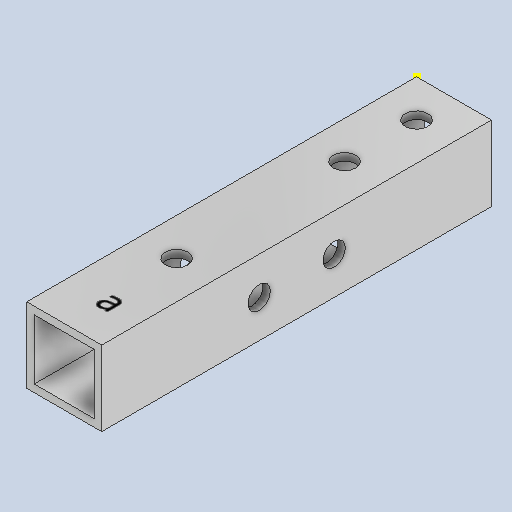
# Autodesk Inventor part: finger_k_mk_2
Saved by Autodesk Inventor 2024.1 (Build 281209000, 209)
## iProperties
Created: 2022-06-23
Part Number: finger_k_mk_2
Material: アルミニウム 6061-AHC
Document SubType Name: Modeling
Designer: zegi
Density: 2.7 g/cm^3
Appearance: アルミニウム - ダーク
Mass: 4.86355 g
Surface Area: 37.6888 cm^2
Volume: 1.80131 cm^3
Author: zegi
Autodesk Inventor part; units mm, degrees
ref_plane "YZ Plane" through (0, 0, 0) normal (1, 0, 0) x (0, 1, 0)
ref_plane "XZ Plane" through (0, 0, 0) normal (0, 1, 0) x (-1, 0, 0)
ref_plane "XY Plane" through (0, 0, 0) normal (0, 0, 1) x (1, 0, 0)
sketch "スケッチ1" plane through (0, 0, 0) normal (0, 0, 1) x (1, 0, 0)
  line L0 (0, 0) -> (10, 0)
  line L1 (10, 0) -> (10, 10)
  line L2 (10, 10) -> (0, 10)
  line L3 (0, 10) -> (0, 0)
  line L4 (1, 9) -> (9, 9)
  line L5 (9, 9) -> (9, 1)
  line L6 (9, 1) -> (1, 1)
  line L7 (1, 1) -> (1, 9)
  dimension "d0" = 10
  dimension "d1" = 10
  dimension "d2" = 1
  constraints: 16 end point, 4 parallel, 2 perpendicular, 1 horizontal, 3 other
  measures "d0" distance of L2.end L1.end
  measures "d1" distance of L1.end L0.end
  measures "d2" distance between parallel lines of L2 L4
extrude "押し出し1" add sketch "スケッチ1" along normal blind 52
sketch "スケッチ2" plane through (0, 10, 0) normal (0, 1, 0) x (1, 0, 0)
  line L0 (10, -52) -> (0, -52) projected
  line L1 (10, 0) -> (10, -52) projected
  line L2 (10, -26) -> (0, -26)
  line L3 (0, 0) -> (0, -52) projected
  point P0 (5, -37)
  point P1 (5, -14.6)
  point P2 (5, -5)
  dimension "d5" = 22.4
  dimension "d7" = 5
  dimension "d8" = 5
  dimension "d35" = 9.6
  dimension "d36" = 11
  constraints: 2 end point, 2 midpoint
  measures "d5" distance of point (5, -14.6) point (5, -37)
  measures "d7" distance from line of L1 point (5, -37)
  measures "d8" distance from line of L1 point (5, -14.6)
  measures "d35" distance of point (5, -5) point (5, -14.6)
  measures "d36" distance from line of L2 point (5, -37)
hole "穴1" at (5, 10, 37) at (5, 10, 14.6) at (5, 10, 5) direction (0, -1, 0) diameter 3 end through all
sketch "スケッチ3" plane through (10, 0, 0) normal (1, 0, 0) x (0, 0, -1)
  line L0 (0, 0) -> (-52, 0) projected
  line L1 (-52, 0) -> (-52, 10) projected
  line L2 (0, 0) -> (-52, 0) projected
  line L3 (-26, 0) -> (-26, 10)
  line L4 (0, 10) -> (-52, 10) projected
  point P0 (-31, 5)
  point P1 (-21, 5)
  dimension "d32" = 5
  dimension "d33" = 5
  constraints: 2 end point, 2 midpoint
  measures "d32" distance from line of point (-21, 5) L3
  measures "d33" distance from line of L3 point (-31, 5)
hole "穴2" at (10, 5, 31) at (10, 5, 21) direction (-1, 0, 0) diameter 3 end through all
sketch "スケッチ4" plane through (0, 10, 0) normal (0, 1, 0) x (1, 0, 0)
  line L0 (4.6245, -45.4744) -> (6.8253, -45.4744) construction
  line L1 (6.8253, -45.4744) -> (6.8253, -52.8345) construction
  line L2 (6.8253, -52.8345) -> (4.6245, -52.8345) construction
  line L3 (4.6245, -52.8345) -> (4.6245, -45.4744) construction
  point P0 (0, 0)
  constraints: 2 other
equation "\"d8\" = d7"
